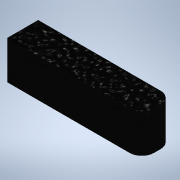
# Autodesk Inventor part: akkum16v
Saved by Autodesk Inventor 2022 (Build 260153000, 153)
## iProperties
Created: 2023-05-26
Part Number: akkum16v
Material: Типовые
Document SubType Name: Modeling
Designer: korsh624
Density: 1 g/cm^3
Appearance: Черный
Author: korsh624
Autodesk Inventor part; units mm, degrees
ref_plane "YZ Plane" through (0, 0, 0) normal (1, 0, 0) x (0, 1, 0)
ref_plane "XZ Plane" through (0, 0, 0) normal (0, 1, 0) x (-1, 0, 0)
ref_plane "XY Plane" through (0, 0, 0) normal (0, 0, 1) x (1, 0, 0)
sketch "Эскиз1" plane through (0, 0, 0) normal (0, 0, 1) x (1, 0, 0)
  line L0 (74.0863, 52.032) -> (-90.9137, 52.032)
  line L1 (-90.9137, 52.032) -> (-90.9137, 5.032)
  line L2 (-90.9137, 5.032) -> (74.0863, 5.032)
  line L3 (74.0863, 5.032) -> (74.0863, 52.032)
  point P0 (0, 0)
  dimension "d0" = 47
  dimension "d1" = 165
  constraints: 8 end point, 2 parallel, 1 horizontal, 1 perpendicular
  measures "d0" distance of L2.end L0.start
  measures "d1" distance of L1.end L2.end
extrude "Выдавливание1" add sketch "Эскиз1" along normal blind 38
fillet "Сопряжение1" radius 15 2 edges at (74.0863, 28.532, 38) (74.0863, 28.532, 0)
